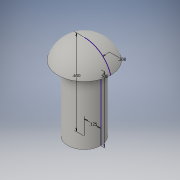
# Autodesk Inventor part: HitchPeg
Saved by Autodesk Inventor 2016 (Build 200138000, 138)
## iProperties
Created: 2018-01-08
Part Number: HitchPeg
Material: Generic
Document SubType Name: Modeling
Designer: sun01147
Density: 1 g/cm^3
Appearance: Default
Author: sun01147
Autodesk Inventor part; units mm, degrees
ref_plane "YZ Plane" through (0, 0, 0) normal (1, 0, 0) x (0, 1, 0)
ref_plane "XZ Plane" through (0, 0, 0) normal (0, 1, 0) x (-1, 0, 0)
ref_plane "XY Plane" through (0, 0, 0) normal (0, 0, 1) x (1, 0, 0)
sketch "Sketch1" plane through (0, 0, 0) normal (0, 0, 1) x (1, 0, 0)
  line L0 (0, 0) -> (3.175, 0)
  line L1 (3.175, 0) -> (3.175, 12.6983)
  line L2 (0, 0) -> (0, 16.51)
  arc A0 (5.0741, 12.6983) -> (0, 16.51) centre (0, 11.2268) ccw
  line L3 (3.175, 12.6983) -> (5.0741, 12.6983)
  dimension "d0" = 3.175
  dimension "d3" = 16.51
  dimension "d5" = 5.2832
  dimension "d8" = 12.6983
  constraints: 8 end point, 2 horizontal, 2 point on circle, 2 vertical, 1 centre point, 1 point on line
  measures "d0" distance of L0.start L0.end
  measures "d3" distance of L0.start L2.end
  measures "d5" radius of A0
  measures "d8" distance of L0.end L1.end
revolve "Revolution1" add sketch "Sketch1" angle 360 about axis through (0, 0, 0) along (0, 1, 0)
body "Solid1"
